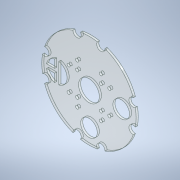
# Autodesk Inventor part: Net_Retainer
Saved by Autodesk Inventor 2020 (Build 240168000, 168)
## iProperties
Created: 2021-06-26
Part Number: Net_Retainer
Material: Glass
Document SubType Name: Modeling
Designer: Workshop
Density: 2.18 g/cm^3
Appearance: Clear
Author: Workshop
Autodesk Inventor part; units mm, degrees
ref_plane "YZ Plane" through (0, 0, 0) normal (1, 0, 0) x (0, 1, 0)
ref_plane "XZ Plane" through (0, 0, 0) normal (0, 1, 0) x (-1, 0, 0)
ref_plane "XY Plane" through (0, 0, 0) normal (0, 0, 1) x (1, 0, 0)
sketch "Sketch1" plane through (0, 0, 0) normal (0, 0, 1) x (1, 0, 0)
  circle A0 centre (-11.4021, -11.4021) radius 1.5 projected
  circle A1 centre (-11.4021, 19.5736) radius 1.5 projected
  circle A2 centre (11.4021, -19.5736) radius 1.5 projected
  circle A3 centre (11.4021, -11.4021) radius 1.5 projected
  circle A4 centre (19.5737, -11.4021) radius 1.5 projected
  circle A5 centre (0, 0) radius 10 projected
  circle A6 centre (11.4021, 11.4021) radius 1.5 projected
  circle A7 centre (19.5736, 11.4021) radius 1.5 projected
  circle A8 centre (11.4021, 19.5737) radius 1.5 projected
  arc A9 (-8.0821, -44.6088) -> (-15.3934, -42.6416) centre (-11.4021, -42.3778) ccw projected
  arc A10 (-8.0821, -44.6088) -> (8.0819, -44.6088) centre (0, 0) ccw projected
  arc A11 (15.3933, -42.6417) -> (8.0819, -44.6088) centre (11.4021, -42.3779) ccw projected
  arc A12 (15.3933, -42.6417) -> (42.6416, -15.3934) centre (0, -0.0002) ccw projected
  arc A13 (44.6088, -8.0821) -> (42.6416, -15.3934) centre (42.3778, -11.4021) ccw projected
  arc A14 (44.6088, -8.0821) -> (44.6088, 8.0819) centre (0, 0) ccw projected
  arc A15 (42.6417, 15.3933) -> (44.6088, 8.0819) centre (42.3779, 11.4021) ccw projected
  arc A16 (42.6417, 15.3933) -> (15.3934, 42.6416) centre (0.0002, 0) ccw projected
  arc A17 (8.0821, 44.6088) -> (15.3934, 42.6416) centre (11.4021, 42.3778) ccw projected
  arc A18 (8.0821, 44.6088) -> (-8.0819, 44.6088) centre (0, 0) ccw projected
  arc A19 (-15.3933, 42.6417) -> (-8.0819, 44.6088) centre (-11.4021, 42.3779) ccw projected
  arc A20 (-15.3933, 42.6417) -> (-42.6416, 15.3934) centre (0, 0.0002) ccw projected
  arc A21 (-44.6088, 8.0821) -> (-42.6416, 15.3934) centre (-42.3778, 11.4021) ccw projected
  arc A22 (-44.6088, 8.0821) -> (-44.6088, -8.0819) centre (0, 0) ccw projected
  arc A23 (-42.6417, -15.3933) -> (-44.6088, -8.0819) centre (-42.3779, -11.4021) ccw projected
  arc A24 (-42.6417, -15.3933) -> (-15.3934, -42.6416) centre (-0.0002, 0) ccw projected
  circle A25 centre (30.9758, 0) radius 8 projected
  circle A26 centre (-11.4021, 11.4021) radius 1.5 projected
  circle A27 centre (-19.5737, 11.4021) radius 1.5 projected
  arc A28 (-28.9758, -9.798) -> (-28.9758, 9.798) centre (-30.9758, 0) ccw projected
  line L0 (-28.9758, 9.798) -> (-28.9758, -9.798) projected
  arc A29 (-40.7737, -2) -> (-32.9758, -9.798) centre (-30.9758, 0) ccw projected
  line L1 (-40.7737, -2) -> (-32.9758, -2) projected
  line L2 (-32.9758, -2) -> (-32.9758, -9.798) projected
  arc A30 (-32.9763, 9.7978) -> (-40.7737, 2) centre (-30.9758, 0) ccw projected
  line L3 (-40.7737, 2) -> (-32.9758, 2) projected
  line L4 (-32.9758, 2) -> (-32.9763, 9.7978) projected
  circle A31 centre (-19.5736, -11.4021) radius 1.5 projected
  circle A32 centre (-11.4021, -19.5737) radius 1.5 projected
  circle A33 centre (0, -30.9758) radius 8 projected
extrude "Extrusion1" add sketch "Sketch1" along normal mid plane 2
body "Solid1"
